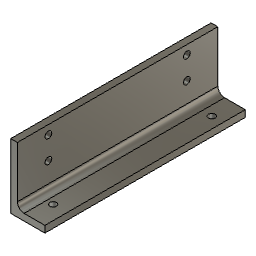
ServoMount v2 (Autodesk Fusion 360 design; units mm, degrees)
Autodesk Fusion 360 part; units mm, degrees
sketch "Sketch1" plane through (0, 0, 0) normal (0, 0, 1) x (1, 0, 0)
  line L0 (0, 0) -> (15.3, 0)
  line L1 (15.3, 0) -> (15.3, 89.7)
  line L2 (15.3, 89.7) -> (0, 89.7)
  line L3 (0, 89.7) -> (0, 0)
  circle A0 centre (9, 10) radius 1.5
  circle A1 centre (10.3, 79.7) radius 1.5
  dimension "d1" = 3
  dimension "d2" = 3
  dimension "d3" = 69.7
  dimension "d4" = 1.3
  dimension "d5" = 10
  dimension "d6" = 10
  dimension "d7" = 9
  dimension "d8" = 5
  constraint horizontal L0
  constraint vertical L1
  constraint horizontal L2
  constraint vertical L3
  constraint coincident L0.start L3.end
  measures "d1" diameter of A0
  measures "d2" diameter of A1
  measures "d3" vertical distance of A0.centre A1.centre
  measures "d4" horizontal distance of A0.centre A1.centre
  measures "d5" distance of L0 A0.centre
  measures "d6" distance of L2 A1.centre
  measures "d7" distance of L3 A0.centre
  measures "d8" distance of L1 A1.centre
extrude "Extrude1" add sketch "Sketch1" along normal blind 3
sketch "Sketch2" plane through (0, 0, 3) normal (0, 0, 1) x (-1, 0, 0)
  circle A0 centre (-10.3, -79.7) radius 1.5
  circle A1 centre (-9, -10) radius 1.5
  line L0 (0, -89.7) -> (0, 0)
  line L1 (0, 0) -> (-15.3, 0)
  line L2 (-15.3, 0) -> (-15.3, -89.7)
  line L3 (-15.3, -89.7) -> (0, -89.7)
  line L4 (0, -89.7) -> (-3, -89.7)
  line L5 (-3, -89.7) -> (-3, 0)
  line L6 (-3, 0) -> (0, 0)
  line L7 (0, 0) -> (0, -89.7)
  dimension "d11" = 3
  constraint horizontal L4
  constraint vertical L5
  constraint horizontal L6
  constraint vertical L7
  constraint coincident L1 L5.end
  constraint coincident L0.start L3.end
  measures "d11" distance of L5 L7
extrude "Extrude2" add sketch "Sketch2" along normal blind 26 contours L0 L1 L3 L4 L5 L6 L7
sketch "Sketch3" plane through (0, 0, 0) normal (-1, 0, 0) x (0, -1, 0)
  line L0 (-89.7, 0) -> (0, 0)
  line L1 (0, 0) -> (0, 29)
  line L2 (0, 29) -> (-89.7, 29)
  line L3 (-89.7, 29) -> (-89.7, 0)
  line L4 (-75.85, 25) -> (-13.85, 25) construction
  line L5 (-13.85, 25) -> (-13.85, 15) construction
  line L6 (-13.85, 15) -> (-75.85, 15) construction
  line L7 (-75.85, 15) -> (-75.85, 25) construction
  line L8 (-44.85, 29) -> (-44.85, 0) construction
  line L9 (-75.85, 20) -> (-13.85, 20) construction
  line L10 (-44.85, 25) -> (-44.85, 15) construction
  circle A0 centre (-75.85, 25) radius 1.5
  circle A1 centre (-13.85, 25) radius 1.5
  circle A2 centre (-13.85, 15) radius 1.5
  circle A3 centre (-75.85, 15) radius 1.5
  dimension "d14" = 62
  dimension "d15" = 10
  dimension "d16" = 4
  dimension "d17" = 3
  dimension "d18" = 3
  dimension "d19" = 3
  dimension "d20" = 3
  constraint horizontal L4
  constraint vertical L5
  constraint horizontal L6
  constraint vertical L7
  constraint midpoint L2 L8.start
  constraint midpoint L0 L8.end
  constraint midpoint L7 L9.start
  constraint midpoint L5 L9.end
  constraint midpoint L4 L10.start
  constraint midpoint L6 L10.end
  constraint collinear L8 L10
  constraint coincident L4.start L7.end
  constraint coincident L4.end L5.start
  constraint coincident L5.end L6.start
  constraint coincident L6.end L7.start
  measures "d14" distance of L5 L7
  measures "d15" distance of L4.start L6.end
  measures "d16" distance of L2 L4
  measures "d17" diameter of A0
  measures "d18" diameter of A1
  measures "d19" diameter of A2
  measures "d20" diameter of A3
extrude "Extrude3" cut sketch "Sketch3" against normal blind 20 contours A0 | A1 | A2 | A3
fillet "Fillet1" radius 3 1 edges at (3, 44.85, 3)
